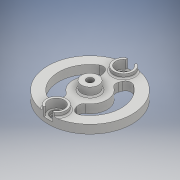
# Autodesk Inventor part: magnet_holder-july21
Saved by Autodesk Inventor 2017 SP1 (Build 210196100, 196)
## iProperties
Part Number: magnet_holder-july21
Material: Générique
Document SubType Name: Modeling
Designer: tmonglon
Density: 1 g/cm^3
Appearance: Par défaut
Author: tmonglon
Autodesk Inventor part; units mm, degrees
ref_plane "YZ Plane" through (0, 0, 0) normal (1, 0, 0) x (0, 1, 0)
ref_plane "XZ Plane" through (0, 0, 0) normal (0, 1, 0) x (-1, 0, 0)
ref_plane "XY Plane" through (0, 0, 0) normal (0, 0, 1) x (1, 0, 0)
sketch "Esquisse1" plane through (0, 0, 0) normal (0, 0, 1) x (1, 0, 0)
  circle A0 centre (0, 0) radius 1.2
  circle A1 centre (0, 0) radius 3
  circle A2 centre (0, 11.8) radius 2
  circle A3 centre (0, 11.8) radius 2.75
  circle A4 centre (0, -11.8) radius 2.75
  circle A5 centre (0, -11.8) radius 2
  circle A6 centre (0, 11.8) radius 1.5
  circle A7 centre (0, -11.8) radius 1.5
  arc A8 (-1.4212, 14.1543) -> (-1.4212, -14.1543) centre (0, 0) ccw
  arc A9 (1.4212, -14.1543) -> (1.4212, 14.1543) centre (0, 0) ccw
  circle A10 centre (0, 0) radius 14.75
  dimension "d1" = 2.4
  dimension "d2" = 6
  dimension "d3" = 4
  dimension "d4" = 11.8
  dimension "d5" = 5.5
  dimension "d8" = 360
  dimension "d12" = 3
  dimension "d15" = 360
  dimension "d95" = 29.5
  constraints: 11 centre point, 8 point on circle, 7 coincident, 14 other
  measures "d1" diameter of A0
  measures "d2" diameter of A1
  measures "d3" diameter of A2
  measures "d4" distance of A2.centre point (0, 0)
  measures "d5" diameter of A3
  measures "d12" diameter of A6
  measures "d95" diameter of A10
extrude "Extrusion10" add sketch "Esquisse1" along normal blind 3 contours A3 A9 A4 A8 | A10
extrude "Extrusion11" add sketch "Esquisse1" along normal blind 6 contours A1
extrude "Extrusion12" add sketch "Esquisse1" along normal blind 0.5 contours A2 | A5
extrude "Extrusion13" add sketch "Esquisse1" along normal blind 1.5 contours A3 | A4
sketch "Esquisse3" plane through (0, 0, 3) normal (0, 0, 1) x (1, 0, 0)
  circle A0 centre (0, 0) radius 1.2 projected
  line L0 (0, 0) -> (-7.6468, 0)
  circle A1 centre (0, 0) radius 3 projected
  line L1 (0, 0) -> (4.4865, 0)
  line L2 (0, 16.0443) -> (0, -15.4592)
  line L3 (0, 0) -> (-3.7622, -10.3366)
  line L4 (0, 0) -> (3.7622, -10.3366)
  line L5 (0, 0) -> (3.7622, 10.3366)
  line L6 (0, 0) -> (-3.7622, 10.3366)
  arc A2 (3.7622, -10.3366) -> (3.7622, 10.3366) centre (0, 0) ccw
  arc A3 (-3.7622, 10.3366) -> (-3.7622, -10.3366) centre (0, 0) ccw
  arc A4 (2.0521, -5.6382) -> (2.0521, 5.6382) centre (0, 0) ccw
  arc A5 (-2.0521, 5.6382) -> (-2.0521, -5.6382) centre (0, 0) ccw
  dimension "d75" = 360
  dimension "d71" = 20
  dimension "d72" = 40
  constraints: 14 end point, 8 point on circle, 5 point on line, 4 centre point, 2 coincident, 1 horizontal, 1 vertical, 11 other
  measures "d71" angle of L3 L2
  measures "d72" angle of L4 L3
extrude "Extrusion15" cut sketch "Esquisse3" against normal through all contours L5 A2 L4 A4 | A5 L3 A3 L6
fillet "Congé1" radius 2 8 edges at (3.7622, -10.3366, 1.5) (-3.7622, -10.3366, 1.5) (-3.7622, 10.3366, 1.5) (3.7622, 10.3366, 1.5) (-2.0521, -5.6382, 1.5) (-2.0521, 5.6382, 1.5) (2.0521, -5.6382, 1.5) (2.0521, 5.6382, 1.5)
chamfer "Chanfrein1" distance 0.5 angle 45 1 edges at (-3, 0, 3)
sketch "Esquisse5" plane through (0, 0, 3) normal (0, 0, 1) x (1, 0, 0)
  circle A0 centre (0, -11.8) radius 1.5 projected
  arc A1 (2.1004, -14.5997) -> (-2.1004, -14.5997) centre (0, -11.8) ccw
  circle A2 centre (0, 11.8) radius 2.75 projected
  arc A3 (-2.1004, 14.5997) -> (2.1004, 14.5997) centre (0, 11.8) ccw
  circle A4 centre (0, -11.8) radius 2.75 projected
  circle A5 centre (0, 11.8) radius 2.75 projected
  circle A6 centre (0, 0) radius 1.2 projected
  circle A7 centre (0, 0) radius 14.75 projected
  arc A8 (-2.1004, -14.5997) -> (2.1004, -14.5997) centre (0, 0) ccw
  arc A9 (2.1004, 14.5997) -> (-2.1004, 14.5997) centre (0, 0) ccw
  circle A10 centre (0, -11.8) radius 2.75 projected
  dimension "d96" = 7
  dimension "d97" = 7
  constraints: 10 point on circle, 4 centre point, 4 coincident
  measures "d96" diameter of A1
  measures "d97" diameter of A3
extrude "Extrusion18" add sketch "Esquisse5" along normal blind 1.5 contours A7 A1 | A7 A3
sketch "Esquisse6" plane through (0, 0, 4.5) normal (0, 0, 1) x (1, 0, 0)
  line L0 (-1.5, -15.5653) -> (1.5, -15.5653)
  line L1 (1.5, -15.5653) -> (1.5, -13.8468)
  line L2 (1.5, -13.8468) -> (-1.5, -13.8468)
  line L3 (-1.5, -13.8468) -> (-1.5, -15.5653)
  line L4 (0, 0) -> (0, -17.5217)
  dimension "d104" = 3
  dimension "d105" = 1.5
  constraints: 10 end point, 2 parallel, 1 horizontal, 1 perpendicular, 1 vertical
  measures "d104" distance of L0.start L0.end
  measures "d105" distance between parallel lines of L4 L3
extrude "Extrusion19" cut sketch "Esquisse6" against normal blind 3
pattern_circular "Réseau circulaire3" count 2 over 360 about axis through (0, 0, 0) along (0, 0, 1) of "Extrusion19"
fillet "Congé3" radius 0.5 2 edges at (0, -8.3, 3) (0, 8.3, 3)
equation "\"d105\" = 0.5 * d104"
